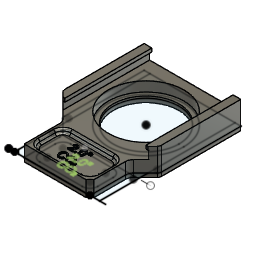
Lens_holder (Autodesk Fusion 360 design; units mm, degrees)
Autodesk Fusion 360 part; units mm, degrees
sketch "Sketch1" plane through (0, 0, 0) normal (0, 1, 0) x (1, 0, 0)
  line L0 (2.5, 0) -> (25, 0)
  line L1 (25, 14.4142) -> (25, 35)
  line L2 (25, 35) -> (0, 35)
  line L3 (0, 35) -> (0, 14.4142)
  line L4 (1.5, 35) -> (1.5, 1)
  line L5 (23.5, 35) -> (23.5, 0)
  circle A0 centre (12.5, 23) radius 9.75
  line L6 (4, 0) -> (20, 0)
  line L7 (21, 1) -> (21, 9.1716)
  line L8 (21, 10) -> (4, 10)
  line L9 (4, 9.1716) -> (4, 0)
  line L10 (21.5858, 10.5858) -> (24.7071, 13.7071)
  line L11 (21, 10) -> (26.6569, 10) construction
  line L12 (3.4142, 10.5858) -> (0.2929, 13.7071)
  line L13 (4, 10) -> (9.6569, 10) construction
  arc A1 (0, 14.4142) -> (0.2929, 13.7071) centre (1, 14.4142) ccw
  arc A2 (24.7071, 13.7071) -> (25, 14.4142) centre (24, 14.4142) ccw
  arc A3 (21.5858, 10.5858) -> (21, 9.1716) centre (23, 9.1716) ccw
  arc A4 (4, 9.1716) -> (3.4142, 10.5858) centre (2, 9.1716) ccw
  line L14 (7, 1) -> (18, 1)
  line L15 (20, 3) -> (20, 7)
  line L16 (18, 9) -> (7, 9)
  line L17 (5, 7) -> (5, 3)
  line L18 (2.5, 0) -> (1.5, 1)
  line L19 (21, 1) -> (20, 0)
  arc A5 (7, 9) -> (5, 7) centre (7, 7) ccw
  arc A6 (5, 3) -> (7, 1) centre (7, 3) ccw
  arc A7 (20, 7) -> (18, 9) centre (18, 7) ccw
  arc A8 (18, 1) -> (20, 3) centre (18, 3) ccw
  line L20 (10.9994, 5.7089) -> (10.9991, 5.4728)
  line L21 (10.9991, 5.4728) -> (9.6771, 5.4744)
  spline S0 degree 2 poles (9.6771, 5.4744) (9.6745, 5.5631) (9.706, 5.6449) knots 0 0 0 1 1 1
  spline S1 degree 2 poles (9.706, 5.6449) (9.7566, 5.7799) (9.868, 5.9107) knots 0 0 0 1 1 1
  spline S2 degree 2 poles (9.868, 5.9107) (9.9793, 6.0416) (10.1896, 6.2132) knots 0 0 0 1 1 1
  spline S3 degree 2 poles (10.1896, 6.2132) (10.516, 6.4802) (10.6308, 6.6363) knots 0 0 0 1 1 1
  spline S4 degree 2 poles (10.6308, 6.6363) (10.7455, 6.7924) (10.7457, 6.9315) knots 0 0 0 1 1 1
  spline S5 degree 2 poles (10.7457, 6.9315) (10.7459, 7.0775) (10.6416, 7.1779) knots 0 0 0 1 1 1
  spline S6 degree 2 poles (10.6416, 7.1779) (10.5374, 7.2783) (10.3696, 7.2785) knots 0 0 0 1 1 1
  spline S7 degree 2 poles (10.3696, 7.2785) (10.1922, 7.2787) (10.0857, 7.1724) knots 0 0 0 1 1 1
  spline S8 degree 2 poles (10.0857, 7.1724) (9.9791, 7.0661) (9.9776, 6.8779) knots 0 0 0 1 1 1
  line L22 (9.9776, 6.8779) -> (9.7252, 6.9041)
  spline S9 degree 2 poles (9.7252, 6.9041) (9.7515, 7.1864) (9.9208, 7.3343) knots 0 0 0 1 1 1
  spline S10 degree 2 poles (9.9208, 7.3343) (10.0901, 7.4821) (10.3753, 7.4818) knots 0 0 0 1 1 1
  spline S11 degree 2 poles (10.3753, 7.4818) (10.6631, 7.4814) (10.8307, 7.3216) knots 0 0 0 1 1 1
  spline S12 degree 2 poles (10.8307, 7.3216) (10.9984, 7.1618) (10.9981, 6.9258) knots 0 0 0 1 1 1
  spline S13 degree 2 poles (10.9981, 6.9258) (10.9979, 6.8057) (10.9487, 6.6898) knots 0 0 0 1 1 1
  spline S14 degree 2 poles (10.9487, 6.6898) (10.8994, 6.5739) (10.7854, 6.4458) knots 0 0 0 1 1 1
  spline S15 degree 2 poles (10.7854, 6.4458) (10.6713, 6.3177) (10.4064, 6.0943) knots 0 0 0 1 1 1
  spline S16 degree 2 poles (10.4064, 6.0943) (10.1852, 5.909) (10.1223, 5.8429) knots 0 0 0 1 1 1
  spline S17 degree 2 poles (10.1223, 5.8429) (10.0595, 5.7768) (10.0185, 5.71) knots 0 0 0 1 1 1
  line L23 (10.0185, 5.71) -> (10.9994, 5.7089)
  line L24 (11.4002, 5.4724) -> (11.4005, 5.752)
  line L25 (11.4005, 5.752) -> (11.6802, 5.7517)
  line L26 (11.6802, 5.7517) -> (11.6799, 5.472)
  line L27 (11.6799, 5.472) -> (11.4002, 5.4724)
  spline S18 degree 2 poles (12.0398, 6.458) (12.0402, 6.8127) (12.1135, 7.0288) knots 0 0 0 1 1 1
  spline S19 degree 2 poles (12.1135, 7.0288) (12.1867, 7.245) (12.3308, 7.3621) knots 0 0 0 1 1 1
  spline S20 degree 2 poles (12.3308, 7.3621) (12.4749, 7.4793) (12.6931, 7.479) knots 0 0 0 1 1 1
  spline S21 degree 2 poles (12.6931, 7.479) (12.8541, 7.4788) (12.9755, 7.4139) knots 0 0 0 1 1 1
  spline S22 degree 2 poles (12.9755, 7.4139) (13.0968, 7.349) (13.1758, 7.2268) knots 0 0 0 1 1 1
  spline S23 degree 2 poles (13.1758, 7.2268) (13.2548, 7.1046) (13.2996, 6.9292) knots 0 0 0 1 1 1
  spline S24 degree 2 poles (13.2996, 6.9292) (13.3444, 6.7539) (13.3441, 6.4564) knots 0 0 0 1 1 1
  spline S25 degree 2 poles (13.3441, 6.4564) (13.3436, 6.1045) (13.2711, 5.8883) knots 0 0 0 1 1 1
  spline S26 degree 2 poles (13.2711, 5.8883) (13.1985, 5.6722) (13.0545, 5.5543) knots 0 0 0 1 1 1
  spline S27 degree 2 poles (13.0545, 5.5543) (12.9104, 5.4365) (12.6907, 5.4367) knots 0 0 0 1 1 1
  spline S28 degree 2 poles (12.6907, 5.4367) (12.4015, 5.4371) (12.2367, 5.6446) knots 0 0 0 1 1 1
  spline S29 degree 2 poles (12.2367, 5.6446) (12.0392, 5.8945) (12.0398, 6.458) knots 0 0 0 1 1 1
  spline S30 degree 2 poles (12.2922, 6.4577) (12.2916, 5.9652) (12.4067, 5.802) knots 0 0 0 1 1 1
  spline S31 degree 2 poles (12.4067, 5.802) (12.5218, 5.6389) (12.691, 5.6387) knots 0 0 0 1 1 1
  spline S32 degree 2 poles (12.691, 5.6387) (12.8601, 5.6385) (12.9756, 5.802) knots 0 0 0 1 1 1
  spline S33 degree 2 poles (12.9756, 5.802) (13.0911, 5.9656) (13.0917, 6.4567) knots 0 0 0 1 1 1
  spline S34 degree 2 poles (13.0917, 6.4567) (13.0922, 6.9506) (12.9772, 7.1131) knots 0 0 0 1 1 1
  spline S35 degree 2 poles (12.9772, 7.1131) (12.8621, 7.2756) (12.6902, 7.2758) knots 0 0 0 1 1 1
  spline S36 degree 2 poles (12.6902, 7.2758) (12.521, 7.276) (12.4199, 7.1328) knots 0 0 0 1 1 1
  spline S37 degree 2 poles (12.4199, 7.1328) (12.2928, 6.9502) (12.2922, 6.4577) knots 0 0 0 1 1 1
  line L28 (13.6746, 6.7616) -> (13.6068, 7.1424)
  line L29 (13.6068, 7.1424) -> (13.6072, 7.4698)
  line L30 (13.6072, 7.4698) -> (13.8868, 7.4695)
  line L31 (13.8868, 7.4695) -> (13.8865, 7.142)
  line L32 (13.8865, 7.142) -> (13.8246, 6.7615)
  line L33 (13.8246, 6.7615) -> (13.6746, 6.7616)
  line L34 (14.1261, 6.7611) -> (14.0597, 7.1418)
  line L35 (14.0597, 7.1418) -> (14.0601, 7.4692)
  line L36 (14.0601, 7.4692) -> (14.3398, 7.4689)
  line L37 (14.3398, 7.4689) -> (14.3394, 7.1415)
  line L38 (14.3394, 7.1415) -> (14.2735, 6.7609)
  line L39 (14.2735, 6.7609) -> (14.1261, 6.7611)
  line L40 (11.2323, 3.0524) -> (11.4969, 2.9852)
  spline S38 degree 2 poles (11.4969, 2.9852) (11.4133, 2.6593) (11.1968, 2.4883) knots 0 0 0 1 1 1
  spline S39 degree 2 poles (11.1968, 2.4883) (10.9804, 2.3173) (10.668, 2.3177) knots 0 0 0 1 1 1
  spline S40 degree 2 poles (10.668, 2.3177) (10.3447, 2.3181) (10.1422, 2.45) knots 0 0 0 1 1 1
  spline S41 degree 2 poles (10.1422, 2.45) (9.9398, 2.5819) (9.8343, 2.8316) knots 0 0 0 1 1 1
  spline S42 degree 2 poles (9.8343, 2.8316) (9.7289, 3.0814) (9.7292, 3.3679) knots 0 0 0 1 1 1
  spline S43 degree 2 poles (9.7292, 3.3679) (9.7296, 3.6803) (9.8493, 3.9128) knots 0 0 0 1 1 1
  spline S44 degree 2 poles (9.8493, 3.9128) (9.9689, 4.1453) (10.1894, 4.2657) knots 0 0 0 1 1 1
  spline S45 degree 2 poles (10.1894, 4.2657) (10.4098, 4.3862) (10.6745, 4.3859) knots 0 0 0 1 1 1
  spline S46 degree 2 poles (10.6745, 4.3859) (10.9746, 4.3856) (11.1791, 4.2325) knots 0 0 0 1 1 1
  spline S47 degree 2 poles (11.1791, 4.2325) (11.3836, 4.0795) (11.4637, 3.8024) knots 0 0 0 1 1 1
  line L41 (11.4637, 3.8024) -> (11.2031, 3.7414)
  spline S48 degree 2 poles (11.2031, 3.7414) (11.1338, 3.9597) (11.0015, 4.0595) knots 0 0 0 1 1 1
  spline S49 degree 2 poles (11.0015, 4.0595) (10.8693, 4.1592) (10.6688, 4.1594) knots 0 0 0 1 1 1
  spline S50 degree 2 poles (10.6688, 4.1594) (10.4382, 4.1597) (10.2832, 4.0494) knots 0 0 0 1 1 1
  spline S51 degree 2 poles (10.2832, 4.0494) (10.1283, 3.9391) (10.0653, 3.7529) knots 0 0 0 1 1 1
  spline S52 degree 2 poles (10.0653, 3.7529) (10.0023, 3.5668) (10.0021, 3.369) knots 0 0 0 1 1 1
  spline S53 degree 2 poles (10.0021, 3.369) (10.0018, 3.1138) (10.0759, 2.9234) knots 0 0 0 1 1 1
  spline S54 degree 2 poles (10.0759, 2.9234) (10.15, 2.733) (10.3068, 2.6387) knots 0 0 0 1 1 1
  spline S55 degree 2 poles (10.3068, 2.6387) (10.4636, 2.5444) (10.6464, 2.5442) knots 0 0 0 1 1 1
  spline S56 degree 2 poles (10.6464, 2.5442) (10.8688, 2.5439) (11.0231, 2.672) knots 0 0 0 1 1 1
  spline S57 degree 2 poles (11.0231, 2.672) (11.1774, 2.8) (11.2323, 3.0524) knots 0 0 0 1 1 1
  spline S58 degree 2 poles (11.7428, 3.3246) (11.7434, 3.8226) (12.0111, 4.104) knots 0 0 0 1 1 1
  spline S59 degree 2 poles (12.0111, 4.104) (12.2789, 4.3854) (12.7018, 4.3849) knots 0 0 0 1 1 1
  spline S60 degree 2 poles (12.7018, 4.3849) (12.9787, 4.3846) (13.2009, 4.252) knots 0 0 0 1 1 1
  spline S61 degree 2 poles (13.2009, 4.252) (13.4232, 4.1194) (13.5395, 3.8825) knots 0 0 0 1 1 1
  spline S62 degree 2 poles (13.5395, 3.8825) (13.6559, 3.6457) (13.6555, 3.3456) knots 0 0 0 1 1 1
  spline S63 degree 2 poles (13.6555, 3.3456) (13.6552, 3.0413) (13.5321, 2.8014) knots 0 0 0 1 1 1
  spline S64 degree 2 poles (13.5321, 2.8014) (13.4091, 2.5614) (13.1838, 2.4382) knots 0 0 0 1 1 1
  spline S65 degree 2 poles (13.1838, 2.4382) (12.9586, 2.315) (12.698, 2.3153) knots 0 0 0 1 1 1
  spline S66 degree 2 poles (12.698, 2.3153) (12.4156, 2.3156) (12.1934, 2.4523) knots 0 0 0 1 1 1
  spline S67 degree 2 poles (12.1934, 2.4523) (11.9712, 2.589) (11.8568, 2.8252) knots 0 0 0 1 1 1
  spline S68 degree 2 poles (11.8568, 2.8252) (11.7425, 3.0613) (11.7428, 3.3246) knots 0 0 0 1 1 1
  spline S69 degree 2 poles (12.0157, 3.3202) (12.0153, 2.9587) (12.2094, 2.7504) knots 0 0 0 1 1 1
  spline S70 degree 2 poles (12.2094, 2.7504) (12.4036, 2.5421) (12.6969, 2.5418) knots 0 0 0 1 1 1
  spline S71 degree 2 poles (12.6969, 2.5418) (12.9957, 2.5414) (13.189, 2.7513) knots 0 0 0 1 1 1
  spline S72 degree 2 poles (13.189, 2.7513) (13.3822, 2.9612) (13.3827, 3.3473) knots 0 0 0 1 1 1
  spline S73 degree 2 poles (13.3827, 3.3473) (13.383, 3.5915) (13.3007, 3.7737) knots 0 0 0 1 1 1
  spline S74 degree 2 poles (13.3007, 3.7737) (13.2183, 3.9559) (13.0595, 4.0564) knots 0 0 0 1 1 1
  spline S75 degree 2 poles (13.0595, 4.0564) (12.9007, 4.1568) (12.7029, 4.1571) knots 0 0 0 1 1 1
  spline S76 degree 2 poles (12.7029, 4.1571) (12.4218, 4.1574) (12.219, 3.9646) knots 0 0 0 1 1 1
  spline S77 degree 2 poles (12.219, 3.9646) (12.0162, 3.7718) (12.0157, 3.3202) knots 0 0 0 1 1 1
  line L42 (14.473, 2.3095) -> (14.4751, 2.1915)
  line L43 (14.4751, 2.1915) -> (13.8142, 2.1798)
  spline S78 degree 2 poles (13.8142, 2.1798) (13.8121, 2.2241) (13.827, 2.2653) knots 0 0 0 1 1 1
  spline S79 degree 2 poles (13.827, 2.2653) (13.8511, 2.3333) (13.9055, 2.3997) knots 0 0 0 1 1 1
  spline S80 degree 2 poles (13.9055, 2.3997) (13.9599, 2.4662) (14.0634, 2.554) knots 0 0 0 1 1 1
  spline S81 degree 2 poles (14.0634, 2.554) (14.224, 2.6906) (14.2799, 2.7697) knots 0 0 0 1 1 1
  spline S82 degree 2 poles (14.2799, 2.7697) (14.3358, 2.8488) (14.3346, 2.9184) knots 0 0 0 1 1 1
  spline S83 degree 2 poles (14.3346, 2.9184) (14.3333, 2.9913) (14.2802, 3.0405) knots 0 0 0 1 1 1
  spline S84 degree 2 poles (14.2802, 3.0405) (14.2272, 3.0897) (14.1433, 3.0882) knots 0 0 0 1 1 1
  spline S85 degree 2 poles (14.1433, 3.0882) (14.0546, 3.0867) (14.0024, 3.0325) knots 0 0 0 1 1 1
  spline S86 degree 2 poles (14.0024, 3.0325) (13.9501, 2.9784) (13.9511, 2.8842) knots 0 0 0 1 1 1
  line L44 (13.9511, 2.8842) -> (13.8247, 2.895)
  spline S87 degree 2 poles (13.8247, 2.895) (13.8351, 3.0364) (13.9184, 3.1119) knots 0 0 0 1 1 1
  spline S88 degree 2 poles (13.9184, 3.1119) (14.0017, 3.1874) (14.1442, 3.1899) knots 0 0 0 1 1 1
  spline S89 degree 2 poles (14.1442, 3.1899) (14.2881, 3.1925) (14.3734, 3.1142) knots 0 0 0 1 1 1
  spline S90 degree 2 poles (14.3734, 3.1142) (14.4587, 3.0359) (14.4608, 2.9179) knots 0 0 0 1 1 1
  spline S91 degree 2 poles (14.4608, 2.9179) (14.4619, 2.8579) (14.4384, 2.7994) knots 0 0 0 1 1 1
  spline S92 degree 2 poles (14.4384, 2.7994) (14.4148, 2.741) (14.359, 2.6759) knots 0 0 0 1 1 1
  spline S93 degree 2 poles (14.359, 2.6759) (14.3032, 2.6108) (14.1729, 2.4966) knots 0 0 0 1 1 1
  spline S94 degree 2 poles (14.1729, 2.4966) (14.0641, 2.4019) (14.0333, 2.3682) knots 0 0 0 1 1 1
  spline S95 degree 2 poles (14.0333, 2.3682) (14.0025, 2.3346) (13.9826, 2.3008) knots 0 0 0 1 1 1
  line L45 (13.9826, 2.3008) -> (14.473, 2.3095)
  circle A9 centre (12.5, 23) radius 8.5
  point P0 (21, 0)
  point P1 (1.5, 0)
  dimension "d1" = 25
  dimension "d2" = 35
  dimension "d3" = 1.5
  dimension "d4" = 1.5
  dimension "d5" = 19.5
  dimension "d6" = 12
  dimension "d7" = 12.5
  dimension "d8" = 17
  dimension "d9" = 4
  dimension "d10" = 10
  dimension "d11" = 45
  dimension "d12" = 135
  dimension "d13" = 1
  dimension "d14" = 2
  dimension "d15" = 2
  dimension "d16" = 15
  dimension "d17" = 1
  dimension "d18" = 8
  dimension "d19" = 1
  dimension "d20" = 1
  dimension "d21" = 1
  dimension "d22" = 1
  dimension "d23" = 1
  dimension "d24" = 2
  dimension "d37" = 17
  constraint horizontal L0
  constraint vertical L1
  constraint horizontal L2
  constraint vertical L3
  constraint coincident L2 L4.start
  constraint perpendicular L0 L4
  constraint coincident L2 L5.start
  constraint coincident L0 L5.end
  constraint perpendicular L0 L5
  constraint horizontal L6
  constraint vertical L7
  constraint horizontal L8
  constraint vertical L9
  constraint coincident L0 L6.start
  constraint horizontal L11
  constraint horizontal L13
  constraint coincident origin L3
  constraint tangent L3 A1
  constraint tangent L12 A1
  constraint coincident L0.end L1
  constraint tangent L10 A2
  constraint tangent L1 A2
  constraint equal A1 A2
  constraint coincident L8.start L7
  constraint coincident L8.start L10
  constraint tangent L7 A3
  constraint tangent L10 A3
  constraint coincident L8.end L12
  constraint coincident L8.end L9
  constraint tangent L12 A4
  constraint tangent L9 A4
  constraint horizontal L14
  constraint vertical L15
  constraint horizontal L16
  constraint vertical L17
  constraint coincident L0 P1
  constraint coincident L4 P1
  constraint coincident origin L0
  constraint coincident P0 L7
  constraint coincident P0 L6
  constraint tangent L16 A5
  constraint tangent L17 A5
  constraint tangent L14 A6
  constraint tangent L17 A6
  constraint equal A5 A6
  constraint tangent L16 A7
  constraint tangent L15 A7
  constraint equal A5 A7
  constraint tangent L14 A8
  constraint tangent L15 A8
  constraint equal A5 A8
  constraint concentric A0 A9
  measures "d1" distance of origin L0.end
  measures "d2" distance of origin L2.end
  measures "d3" distance of L3 L4
  measures "d4" distance of L1 L5
  measures "d5" diameter of A0
  measures "d6" distance of L2 A0.centre
  measures "d7" distance of L1 A0.centre
  measures "d8" distance of L7 L9
  measures "d9" distance of L1 L7
  measures "d10" distance of L6 L8
  measures "d11" angle of L10 L11
  measures "d12" angle of L12 L13
  measures "d13" radius of A1
  measures "d14" radius of A3
  measures "d15" radius of A4
  measures "d16" distance of L15 L17
  measures "d17" distance of L7 L15
  measures "d18" distance of L14 L16
  measures "d19" distance of L0 L14
  measures "d20" distance of L0.start P1
  measures "d21" distance of L4.end P1
  measures "d22" distance of P0 L7.start
  measures "d23" distance of P0 L6.end
  measures "d24" radius of A5
  measures "d37" diameter of A9
extrude "Extrude1" add sketch "Sketch1" along normal blind 3 contours L0 L2 L4 L5 L6 L7 L9 L10 L12 A3 A4 L19 | L2 L3 L4 L12 A1 | L1 L2 L5 L10 A2
extrude "Extrude2" add sketch "Sketch1" along normal blind 2 contours L14 L15 L16 L17 A5 A6 A7 A8 | L20 L21 S0 S1 S2 S3 S4 S5 S6 S7 S8 L22 S9 S10 S11 S12 S13 S14 S15 S16 S17 L23 | L24 L25 L26 L27 | S18 S19 S20 S21 S22 S23 S24 S25 S26 S27 S28 S29 | S30 S31 S32 S33 S34 S35 S36 S37 | L28 L29 L30 L31 L32 L33 | L34 L35 L36 L37 L38 L39 | L40 S38 S39 S40 S41 S42 S43 S44 S45 S46 S47 L41 S48 S49 S50 S51 S52 S53 S54 S55 S56 S57 | S58 S59 S60 S61 S62 S63 S64 S65 S66 S67 S68 | S69 S70 S71 S72 S73 S74 S75 S76 S77 | L42 L43 S78 S79 S80 S81 S82 S83 S84 S85 S86 L44 S87 S88 S89 S90 S91 S92 S93 S94 S95 L45
extrude "Extrude3" add sketch "Sketch1" along normal blind 2.25 contours L20 L21 S0 S1 S2 S3 S4 S5 S6 S7 S8 L22 S9 S10 S11 S12 S13 S14 S15 S16 S17 L23 | L24 L25 L26 L27 | S18 S19 S20 S21 S22 S23 S24 S25 S26 S27 S28 S29 | L28 L29 L30 L31 L32 L33 | L34 L35 L36 L37 L38 L39 | L40 S38 S39 S40 S41 S42 S43 S44 S45 S46 S47 L41 S48 S49 S50 S51 S52 S53 S54 S55 S56 S57 | S58 S59 S60 S61 S62 S63 S64 S65 S66 S67 S68 | L42 L43 S78 S79 S80 S81 S82 S83 S84 S85 S86 L44 S87 S88 S89 S90 S91 S92 S93 S94 S95 L45
fillet "Fillet1" radius 0.5 8 edges at (20, 2, -5) (19.4142, 2, -1.5858) (12.5, 2, -1) (5.5858, 2, -1.5858) (5, 2, -5) (5.5858, 2, -8.4142) (12.5, 2, -9) (19.4142, 2, -8.4142)
fillet "Fillet1" radius 0.5 8 edges at (20, 3, -5) (19.4142, 3, -1.5858) (12.5, 3, -1) (5.5858, 3, -1.5858) (5, 3, -5) (5.5858, 3, -8.4142) (12.5, 3, -9) (19.4142, 3, -8.4142)
extrude "Extrude4" add sketch "Sketch1" along normal blind 0.5 and the other way blind 1 contours A0
move_face "OffsetFaces1" offset 1 1 faces at (11.0044, -0.6667, -13.3654)
extrude "Extrude5" add sketch "Sketch1" along normal blind 6 contours L2 L3 L4 L12 A1 | L1 L2 L5 L10 A2
extrude "Extrude6" add 1 faces at (1.5, 5, -27.5) along direction (1, 0, 0) blind 0.5
extrude "Extrude7" add 1 faces at (23.5, 5, -27.5) along direction (-1, 0, 0) blind 0.5
sketch "Sketch2" plane through (0, 0, -35) normal (0, 0, -1) x (-1, 0, 0)
  line L0 (-25, 0) -> (0, 0)
  line L1 (0, 0) -> (0, 6)
  line L2 (0, 6) -> (-2, 6)
  line L3 (-2, 6) -> (-2, 3)
  line L4 (-2, 3) -> (-23, 3)
  line L5 (-23, 3) -> (-23, 6)
  line L6 (-23, 6) -> (-25, 6)
  line L7 (-25, 6) -> (-25, 0)
  line L8 (-2, 3) -> (-1.4, 3)
  line L9 (-1.4, 3) -> (-1.4, 5.1)
  line L10 (-1.4, 5.1) -> (-2, 5.1)
  line L11 (-2, 5.1) -> (-2, 3)
  line L12 (-12.5, 0) -> (-12.5, 3)
  line L13 (-23.6, 3) -> (-23.6, 5.1)
  line L14 (-23.6, 5.1) -> (-23, 5.1)
  line L15 (-23, 3) -> (-23.6, 3)
  line L16 (-23, 5.1) -> (-23, 3)
  dimension "d49" = 0.9
  dimension "d50" = 1.4
  constraint horizontal L8
  constraint vertical L9
  constraint horizontal L10
  constraint vertical L11
  constraint coincident L3.end L4.start
  constraint midpoint L0 L12.start
  constraint midpoint L4 L12.end
  constraint symmetric L3.end L12 L4.end
  constraint symmetric L8.end L12 L13.start
  constraint symmetric L9.end L12 L13.end
  constraint symmetric L10.end L12 L14.end
  measures "d49" distance of L2 L10
  measures "d50" distance of L1 L9
extrude "Extrude8" cut sketch "Sketch2" against normal blind 23 contours L3 L8 L9 L10 L11 | L5 L13 L14 L15 L16
sketch "Sketch3" plane through (0, 0, 0) normal (0, -1, 0) x (1, 0, 0)
  circle A0 centre (12.5, -23) radius 10.75
  line L0 (24.7071, -13.7071) -> (21.5858, -10.5858)
  arc A1 (21, -9.1716) -> (21.5858, -10.5858) centre (23, -9.1716) ccw
  line L1 (21, -9.1716) -> (21, -1)
  line L2 (21, -1) -> (20, 0)
  line L3 (20, 0) -> (4, 0)
  line L4 (4, 0) -> (4, -9.1716)
  arc A2 (3.4142, -10.5858) -> (4, -9.1716) centre (2, -9.1716) ccw
  line L5 (3.4142, -10.5858) -> (0.2929, -13.7071)
  arc A3 (0.2929, -13.7071) -> (0, -14.4142) centre (1, -14.4142) ccw
  line L6 (0, -14.4142) -> (0, -35)
  line L7 (0, -35) -> (25, -35)
  line L8 (25, -35) -> (25, -14.4142)
  arc A4 (25, -14.4142) -> (24.7071, -13.7071) centre (24, -14.4142) ccw
  circle A5 centre (12.5, -23) radius 11
  dimension "d53" = 22
  constraint concentric A0 A5
  measures "d53" diameter of A5
extrude "Extrude9" add sketch "Sketch3" along normal blind 1 contours L0 A1 L1 L2 L3 L4 A2 L5 A3 L6 L7 L8 A4
chamfer "Chamfer1" distance 1 angle 45 2 edges at (2.2444, -1, -19.0222) (2.4775, -1, -26.8874)
equation "d21 = d20"
equation "d23 = d22"
